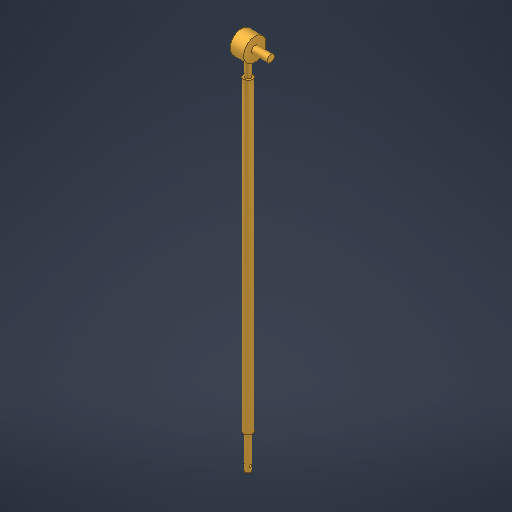
# Autodesk Inventor part: tierod
Saved by Autodesk Inventor 2026.2 (Build 302298010, 298A)
## iProperties
Created: 2026-07-06
Part Number: tierod
Material: Generic
Document SubType Name: Modeling
Designer: tasle
Density: 1 g/cm^3
Appearance: Default
Author: tasle
Autodesk Inventor part; units mm, degrees
ref_plane "YZ Plane" through (0, 0, 0) normal (1, 0, 0) x (0, 1, 0)
ref_plane "XZ Plane" through (0, 0, 0) normal (0, 1, 0) x (-1, 0, 0)
ref_plane "XY Plane" through (0, 0, 0) normal (0, 0, 1) x (1, 0, 0)
sketch "Sketch1" plane through (0, 0, 0) normal (1, 0, 0) x (0, 1, 0)
  line L0 (300, 0) -> (-300, 0)
  circle A0 centre (287.5, 0) radius 12.5
  circle A1 centre (287.5, 0) radius 4
  line L1 (287.5, 0) -> (-120, 0)
  line L2 (-120, 0) -> (-120, 3)
  line L3 (-120, 3) -> (287.5, 3)
  line L4 (287.5, 3) -> (287.5, 0)
  line L5 (257.5, 0) -> (-82.5, 0)
  line L6 (-82.5, 0) -> (-82.5, 5)
  line L7 (-82.5, 5) -> (257.5, 5)
  line L8 (257.5, 5) -> (257.5, 0)
  point P0 (0, 0)
  point P1 (-120, 0)
  point P2 (283.5, 0)
  point P3 (284.8542, 3)
  point P4 (-82.5, 0)
  point P5 (257.5, 0)
  dimension "d0" = 600
  dimension "d1" = 25
  dimension "d2" = 12.5
  dimension "d3" = 8
  dimension "d4" = 3
  dimension "d12" = 340
  dimension "d13" = 5
  dimension "d16" = 30
  constraints: 18 end point, 4 parallel, 3 horizontal, 2 centre point, 2 perpendicular, 2 point on line, 1 coincident, 1 midpoint
  measures "d0" distance of L0.start L0.end
  measures "d1" diameter of A0
  measures "d2" distance of L0.start A0.centre
  measures "d3" diameter of A1
  measures "d4" distance of L1.end L2.end
  measures "d12" distance of L6.end L7.end
  measures "d13" distance of L5.end L6.end
  measures "d16" distance from line of A0.centre L8
revolve "Revolution1" add sketch "Sketch1" angle 360 about axis through (0, 300, 0) along (0, -1, 0) picked at (277.9311, 1.2871) contours L3 A1 L0 A0 | A0 L0 L8 L3 | L8 L0 L6 L3 | L6 L0 L2 L3
extrude "Extrusion2" add sketch "Sketch1" along normal blind 25 contours A1 L0 | L0 L4 L3 A1 | L0 A1 L3 L4
extrude "Extrusion3" add sketch "Sketch1" along normal mid plane 15 contours A0 L0 A1 | L0 A1 L3 A0 | A1 L0 | L0 L4 L3 A1 | L3 A1 L0 A0 | L0 A1 L3 L4
revolve "Revolution2" add sketch "Sketch1" angle 360 about axis through (0, 287.5, 0) along (0, -1, 0) contours L8 L0 L6 L3 | L3 L6 L7 L8
sketch "Sketch2" plane through (0, 0, 0) normal (1, 0, 0) x (0, 1, 0)
  circle A0 centre (-114.1043, 0) radius 1.5
  point P0 (0, 0)
  dimension "d17" = 3
  constraints: 1 centre point
  measures "d17" diameter of A0
extrude "Extrusion4" cut sketch "Sketch2" along normal mid plane 15
body "Solid1"
